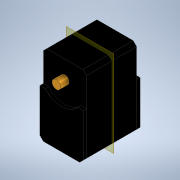
# Autodesk Inventor part: feetech_sc215
Saved by Autodesk Inventor 2020.1 (Build 241239000, 239)
## iProperties
Created: 2019-11-19
Part Number: feetech_sc215
Material: Generic
Document SubType Name: Modeling
Designer: 19Bar
Density: 1 g/cm^3
Appearance: Default
Author: 19Bar
Autodesk Inventor part; units mm, degrees
ref_plane "YZ Plane" through (0, 0, 0) normal (1, 0, 0) x (0, 1, 0)
ref_plane "XZ Plane" through (0, 0, 0) normal (0, 1, 0) x (-1, 0, 0)
ref_plane "XY Plane" through (0, 0, 0) normal (0, 0, 1) x (1, 0, 0)
sketch "Sketch1" plane through (0, 0, 0) normal (0, 0, 1) x (1, 0, 0)
  line L0 (0, 0) -> (25, 0)
  line L1 (25, 0) -> (25, 45.5)
  line L2 (25, 45.5) -> (0, 45.5)
  line L3 (0, 45.5) -> (0, 0)
  dimension "d0" = 25
  dimension "d1" = 45.5
  constraints: 8 end point, 2 parallel, 1 horizontal, 1 perpendicular
  measures "d0" distance of L2.end L1.end
  measures "d1" distance of L1.end L0.end
extrude "Extrusion1" add sketch "Sketch1" along normal blind 29
chamfer "Chamfer1" distance 2 angle 45 4 edges at (25, 45.5, 14.5) (0, 45.5, 14.5) (25, 0, 14.5) (0, 0, 14.5)
sketch "Sketch2" plane through (0, 0, 29) normal (0, 0, 1) x (1, 0, 0)
  line L0 (23, 45.5) -> (2, 45.5) projected
  line L1 (12.5, 45.5) -> (12.5, 0)
  line L2 (2, 0) -> (23, 0) projected
  line L3 (12.5, 22.75) -> (12.5, 35.25)
  circle A0 centre (12.5, 35.25) radius 12.5
  line L4 (12.5, 0) -> (2, 0)
  line L5 (0, 2) -> (2, 0) projected
  line L6 (2, 0) -> (0, 1.9914)
  line L7 (0, 1.9914) -> (0, 26.9914)
  line L8 (0, 43.5) -> (0, 2) projected
  line L9 (0, 26.9914) -> (3.1167, 26.9914)
  line L10 (12.5, 0) -> (23, 0)
  line L11 (23, 0) -> (24.9828, 1.9914)
  line L12 (24.9828, 1.9914) -> (23, 0)
  line L13 (24.9828, 1.9914) -> (25, 26.9914)
  line L14 (25, 2) -> (25, 43.5) projected
  line L15 (25, 26.9914) -> (21.8833, 26.9914)
  point P0 (0, 0)
  dimension "d8" = 12.5
  dimension "d9" = 25
  dimension "d10" = 25
  constraints: 22 end point, 4 point on line, 3 midpoint, 3 point on circle, 2 collinear, 2 perpendicular, 1 centre point, 1 coincident, 1 horizontal
  measures "d8" distance of L3.start L3.end
  measures "d9" distance of L6.end L7.end
  measures "d10" distance of L11.end L13.end
extrude "Extrusion2" add sketch "Sketch2" along normal blind 2 contours L15 L13 L11 L2 L1 A0 | L1 L2 L5 L7 L9 A0
ref_plane "Work Plane1" through (0, 0, 14.5) normal (0, 0, 1) x (1, 0, 0)
sketch "Sketch3" plane through (0, 0, 29) normal (0, 0, 1) x (1, 0, 0)
  arc A0 (3.1167, 26.9914) -> (21.8833, 26.9914) centre (12.5, 35.25) ccw projected
  circle A1 centre (12.5, 35.25) radius 2.5
  point P0 (0, 0)
  dimension "d13" = 5
  constraints: 1 centre point, 1 coincident
  measures "d13" diameter of A1
extrude "Extrusion3" add sketch "Sketch3" along normal blind 5
mirror "Mirror1" about plane through (0, 0, 14.5) normal (0, 0, 1) of "Extrusion2", "Extrusion3"
sketch "Sketch5" plane through (12.5, 35.25, -2) normal (0, 0, -1) x (-1, 0, 0)
  circle A0 centre (0, 0) radius 2.5 projected
  line L0 (0, 0) -> (0, -13)
  line L1 (0, -13) -> (10, -13)
  line L2 (10, -13) -> (10, -18)
  line L3 (10, -18) -> (-10, -18)
  line L4 (-10, -18) -> (-10, -13)
  line L5 (-10, -13) -> (0, -13)
  point P0 (12.5, -35.25)
  dimension "d16" = 13
  dimension "d17" = 10
  dimension "d18" = 5
  dimension "d19" = 20
  constraints: 12 end point, 5 perpendicular, 1 point on line, 1 vertical
  measures "d16" distance of L0.start L0.end
  measures "d17" distance of L0.end L1.end
  measures "d18" distance of L1.end L2.end
  measures "d19" distance of L2.end L3.end
extrude "Extrusion4" cut sketch "Sketch5" against normal blind 5 contours L1 L2 L3 L4 L5
ref_plane "Work Plane2" through (0, 0, 14.5) normal (0, 0, 1) x (1, 0, 0)
body "Solid1"
